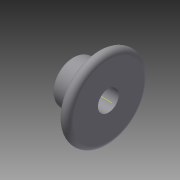
# Autodesk Inventor part: revolution_example
Saved by Autodesk Inventor 2015 (Build 190159000, 159)
## iProperties
Created: 2015-02-06
Part Number: revolution_example
Material: Generic
Document SubType Name: Modeling
Designer: admin
Density: 1 g/cm^3
Appearance: Default
Author: admin
Autodesk Inventor part; units mm, degrees
ref_plane "YZ Plane" through (0, 0, 0) normal (1, 0, 0) x (0, 1, 0)
ref_plane "XZ Plane" through (0, 0, 0) normal (0, 1, 0) x (-1, 0, 0)
ref_plane "XY Plane" through (0, 0, 0) normal (0, 0, 1) x (1, 0, 0)
sketch "Sketch1" plane through (0, 0, 0) normal (0, 1, 0) x (-1, 0, 0)
  line L0 (10.0011, -4.0004) -> (-4.061, -4.0004)
  line L1 (-4.061, -4.0004) -> (-4.061, -20.083)
  line L2 (-4.061, -20.083) -> (0, -13.9813)
  line L3 (0, -13.9813) -> (0, -8.1221)
  line L4 (0, -8.1221) -> (10.0011, -8.1221)
  line L5 (10.0011, -8.1221) -> (10.0011, -4.0004)
  line L6 (12.8135, 0) -> (-6.8735, 0) projected
  point P0 (0, 0)
  constraints: 12 end point, 3 perpendicular, 1 horizontal, 1 parallel
revolve "Revolution1" add sketch "Sketch1" angle 360 about axis through (-10, 0, 0) along (1, 0, 0)
fillet "Fillet1" radius 2 1 edges at (4.061, 0, 20.083)
fillet "Fillet2" radius 2 2 edges at (-10.0011, 0, 8.1221) (0, 0, 8.1221)
body "Solid1"
